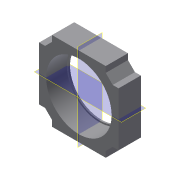
# Autodesk Inventor part: 20_Cube_Insert_VCM_MirrorMount_KES400A
Saved by Autodesk Inventor 2019.4 (Build 234330000, 330)
## iProperties
Created: 2019-10-23
Part Number: 20_Cube_Insert_VCM_MirrorMount_KES400A
Material: Generic
Document SubType Name: Modeling
Designer: marsikovabarbora
Density: 1 g/cm^3
Appearance: Default
Lens_diameter: 25,400 mm
Author: marsikovabarbora
Autodesk Inventor part; units mm, degrees
ref_plane "YZ Plane" through (0, 0, 0) normal (1, 0, 0) x (0, 1, 0)
ref_plane "XZ Plane" through (0, 0, 0) normal (0, 1, 0) x (-1, 0, 0)
ref_plane "XY Plane" through (0, 0, 0) normal (0, 0, 1) x (1, 0, 0)
sketch "Sketch1" plane through (0, 0, 0) normal (0, 0, 1) x (1, 0, 0)
  line L0 (-37.8611, 0) -> (52.8619, 0) construction
  line L1 (0, -34.8609) -> (0, 34.8609) construction
  line L2 (0, 0) -> (13.4339, 13.4339) construction
  line L3 (0, 0) -> (18.9985, 0) construction
  line L4 (0, 24.9006) -> (16.8, 24.9006)
  line L5 (16.8, 24.9006) -> (16.8, 21.2406)
  line L6 (16.8, 21.2406) -> (19.0203, 19.0203)
  line L7 (24.9006, 0) -> (24.9006, 16.8)
  line L8 (24.9006, 16.8) -> (21.2406, 16.8)
  line L9 (21.2406, 16.8) -> (19.0203, 19.0203)
  line L10 (0, 0) -> (-13.4339, 13.4339) construction
  line L11 (0, 0) -> (-18.9985, 0) construction
  line L12 (0, 24.9006) -> (-16.8, 24.9006)
  line L13 (-16.8, 24.9006) -> (-16.8, 21.2406)
  line L14 (-16.8, 21.2406) -> (-19.0203, 19.0203)
  line L15 (-24.9006, 0) -> (-24.9006, 16.8)
  line L16 (-24.9006, 16.8) -> (-21.2406, 16.8)
  line L17 (-21.2406, 16.8) -> (-19.0203, 19.0203)
  line L18 (0, 0) -> (13.4339, -13.4339) construction
  line L19 (0, -24.9006) -> (16.8, -24.9006)
  line L20 (16.8, -24.9006) -> (16.8, -21.2406)
  line L21 (16.8, -21.2406) -> (19.0203, -19.0203)
  line L22 (24.9006, 0) -> (24.9006, -16.8)
  line L23 (24.9006, -16.8) -> (21.2406, -16.8)
  line L24 (21.2406, -16.8) -> (19.0203, -19.0203)
  line L25 (0, 0) -> (-13.4339, -13.4339) construction
  line L26 (0, -24.9006) -> (-16.8, -24.9006)
  line L27 (-16.8, -24.9006) -> (-16.8, -21.2406)
  line L28 (-16.8, -21.2406) -> (-19.0203, -19.0203)
  line L29 (-24.9006, 0) -> (-24.9006, -16.8)
  line L30 (-24.9006, -16.8) -> (-21.2406, -16.8)
  line L31 (-21.2406, -16.8) -> (-19.0203, -19.0203)
  circle A0 centre (37.4, 10.6752) radius 1 projected
  circle A1 centre (30.9, -9.8248) radius 1 projected
  line L32 (39.9015, 13.4339) -> (24.9006, 13.4339)
  line L33 (24.9006, 13.4339) -> (24.9006, -12.4218)
  line L34 (24.9006, -12.4218) -> (39.9015, -12.4218)
  line L35 (39.9015, -12.4218) -> (39.9015, 13.4339)
  dimension "d0" = 45
  dimension "d1" = 3.14
  dimension "d2" = 3.66
  dimension "d3" = 16.8
  constraints: 68 end point, 24 symmetric about line, 6 point on line, 3 horizontal, 3 perpendicular, 2 parallel, 1 equal length
  measures "d0" angle of L3 L2
  measures "d1" distance of L5.end L6.end
  measures "d2" distance of L4.end L5.end
  measures "d3" distance of L4.start L4.end
extrude "Thickness" add sketch "Sketch1" along normal blind 14 contours L4 L5 L6 L9 L8 L7 L22 L23 L24 L21 L20 L19 L26 L27 L28 L31 L30 L29 L15 L16 L17 L14 L13 L12 | L32 L35 L34 L22 L7 | A0 | A1
sketch "Sketch3" plane through (0, 0, 0) normal (0, 0, -1) x (-1, 0, 0)
  line L0 (-16.8, 24.9006) -> (16.8, 24.9006) projected
  line L1 (16.8, 24.9006) -> (16.8, 21.2406) projected
  line L2 (16.8, 21.2406) -> (21.2406, 16.8) projected
  line L3 (21.2406, 16.8) -> (24.9006, 16.8) projected
  line L4 (24.9006, 16.8) -> (24.9006, -16.8) projected
  line L5 (24.9006, -16.8) -> (21.2406, -16.8) projected
  line L6 (21.2406, -16.8) -> (16.8, -21.2406) projected
  line L7 (16.8, -21.2406) -> (16.8, -24.9006) projected
  line L8 (16.8, -24.9006) -> (-16.8, -24.9006) projected
  line L9 (-16.8, -24.9006) -> (-16.8, -21.2406) projected
  line L10 (-16.8, -21.2406) -> (-21.2406, -16.8) projected
  line L11 (-21.2406, -16.8) -> (-24.9006, -16.8) projected
  line L12 (-24.9006, -16.8) -> (-24.9006, -12.4218) projected
  line L13 (-24.9006, 16.8) -> (-21.2406, 16.8) projected
  line L14 (-21.2406, 16.8) -> (-16.8, 21.2406) projected
  line L15 (-16.8, 21.2406) -> (-16.8, 24.9006) projected
  line L16 (16.8994, 25) -> (-16.8994, 25)
  line L17 (-16.8994, 25) -> (-16.8994, 21.2818)
  line L18 (-16.8994, 21.2818) -> (-21.2818, 16.8994)
  line L19 (-21.2818, 16.8994) -> (-25, 16.8994)
  line L20 (-25, 16.8994) -> (-25, -16.8994)
  line L21 (-25, -16.8994) -> (-21.2818, -16.8994)
  line L22 (-21.2818, -16.8994) -> (-16.8994, -21.2818)
  line L23 (-16.8994, -21.2818) -> (-16.8994, -25)
  line L24 (-16.8994, -25) -> (16.8994, -25)
  line L25 (16.8994, -25) -> (16.8994, -21.2818)
  line L26 (16.8994, -21.2818) -> (21.2818, -16.8994)
  line L27 (21.2818, -16.8994) -> (25, -16.8994)
  line L28 (25, -16.8994) -> (25, 16.8994)
  line L29 (25, 16.8994) -> (21.2818, 16.8994)
  line L30 (21.2818, 16.8994) -> (16.8994, 21.2818)
  line L31 (16.8994, 21.2818) -> (16.8994, 25)
  line L32 (-39.9015, 13.4339) -> (-24.9006, 13.4339) projected
  line L33 (-24.9006, 13.4339) -> (-24.9006, 16.8) projected
  line L34 (-24.9006, -12.4218) -> (-39.9015, -12.4218) projected
  line L35 (-39.9015, -12.4218) -> (-39.9015, 13.4339) projected
  point P0 (0, 0)
  dimension "d22" = 50
  constraints: 32 end point, 15 other
  measures "d22" distance between parallel lines of L20 L28
extrude "Extrusion3" add sketch "Sketch3" against normal up to surface (14 mm away)
ref_plane "Work Plane1" through (0, -16.8994, 0) normal (-1, 0, 0) x (0, 0, 1)
ref_plane "Work Plane2" through (-16.8994, 0, 0) normal (0, -1, 0) x (1, 0, 0)
sketch "Sketch4" plane through (0, 0, 0) normal (0, 0, -1) x (-1, 0, 0)
  arc A0 (12.7755, -29.7) -> (13.7755, -30.7) centre (13.7755, -29.7) ccw projected
  line L0 (13.7755, -30.7) -> (16.92, -30.7) projected
  line L1 (16.92, -30.7) -> (16.92, -5) projected
  line L2 (16.92, -5) -> (7.3923, -5) projected
  arc A1 (7.3923, -5) -> (6.3923, -6) centre (7.3923, -6) ccw projected
  line L3 (6.3923, -6) -> (6.3923, -7.8624) projected
  arc A2 (5.3923, -8.8624) -> (6.3923, -7.8624) centre (5.3923, -7.8624) ccw projected
  line L4 (5.3923, -8.8624) -> (-13.08, -8.8624) projected
  line L5 (-13.08, -8.8624) -> (-13.08, -20.397) projected
  arc A3 (-14.08, -21.397) -> (-13.08, -20.397) centre (-14.08, -20.397) ccw projected
  line L6 (-14.08, -21.397) -> (-15.08, -21.397) projected
  arc A4 (-15.08, -21.397) -> (-16.08, -22.397) centre (-15.08, -22.397) ccw projected
  line L7 (-16.08, -22.397) -> (-16.08, -24.9624) projected
  arc A5 (-16.08, -24.9624) -> (-15.08, -25.9624) centre (-15.08, -24.9624) ccw projected
  line L8 (-15.08, -25.9624) -> (11.7755, -25.9624) projected
  arc A6 (12.7755, -26.9624) -> (11.7755, -25.9624) centre (11.7755, -26.9624) ccw projected
  line L9 (12.7755, -26.9624) -> (12.7755, -29.7) projected
  line L10 (4.42, -24) -> (-11.08, -24) projected
  line L11 (-11.08, -24) -> (-11.08, -10.5) projected
  line L12 (-11.08, -10.5) -> (4.42, -10.5) projected
  line L13 (4.42, -10.5) -> (4.42, -24) projected
  circle A7 centre (14.42, -28) radius 1 projected
  circle A8 centre (7.92, -7.5) radius 1 projected
  circle A9 centre (-13.58, -23) radius 1 projected
  arc A10 (12.7755, 5.3) -> (13.7755, 4.3) centre (13.7755, 5.3) ccw projected
  line L14 (13.7755, 4.3) -> (16.92, 4.3) projected
  line L15 (16.92, 4.3) -> (16.92, 30) projected
  line L16 (16.92, 30) -> (7.3923, 30) projected
  arc A11 (7.3923, 30) -> (6.3923, 29) centre (7.3923, 29) ccw projected
  line L17 (6.3923, 29) -> (6.3923, 27.1376) projected
  arc A12 (5.3923, 26.1376) -> (6.3923, 27.1376) centre (5.3923, 27.1376) ccw projected
  line L18 (5.3923, 26.1376) -> (-13.08, 26.1376) projected
  line L19 (-13.08, 26.1376) -> (-13.08, 14.603) projected
  arc A13 (-14.08, 13.603) -> (-13.08, 14.603) centre (-14.08, 14.603) ccw projected
  line L20 (-14.08, 13.603) -> (-15.08, 13.603) projected
  arc A14 (-15.08, 13.603) -> (-16.08, 12.603) centre (-15.08, 12.603) ccw projected
  line L21 (-16.08, 12.603) -> (-16.08, 10.0376) projected
  arc A15 (-16.08, 10.0376) -> (-15.08, 9.0376) centre (-15.08, 10.0376) ccw projected
  line L22 (-15.08, 9.0376) -> (11.7755, 9.0376) projected
  arc A16 (12.7755, 8.0376) -> (11.7755, 9.0376) centre (11.7755, 8.0376) ccw projected
  line L23 (12.7755, 8.0376) -> (12.7755, 5.3) projected
  line L24 (4.42, 11) -> (-11.08, 11) projected
  line L25 (-11.08, 11) -> (-11.08, 24.5) projected
  line L26 (-11.08, 24.5) -> (4.42, 24.5) projected
  line L27 (4.42, 24.5) -> (4.42, 11) projected
  circle A17 centre (14.42, 7) radius 1 projected
  circle A18 centre (7.92, 27.5) radius 1 projected
  circle A19 centre (-13.58, 12) radius 1 projected
  arc A20 (-35.7555, 12.3752) -> (-36.7555, 13.3752) centre (-36.7555, 12.3752) ccw projected
  line L28 (-36.7555, 13.3752) -> (-39.9, 13.3752) projected
  line L29 (-39.9, 13.3752) -> (-39.9, -12.3248) projected
  line L30 (-39.9, -12.3248) -> (-30.3723, -12.3248) projected
  arc A21 (-30.3723, -12.3248) -> (-29.3723, -11.3248) centre (-30.3723, -11.3248) ccw projected
  line L31 (-29.3723, -11.3248) -> (-29.3723, -9.4624) projected
  arc A22 (-28.3723, -8.4624) -> (-29.3723, -9.4624) centre (-28.3723, -9.4624) ccw projected
  line L32 (-28.3723, -8.4624) -> (-9.9, -8.4624) projected
  line L33 (-9.9, -8.4624) -> (-9.9, 3.0723) projected
  arc A23 (-8.9, 4.0723) -> (-9.9, 3.0723) centre (-8.9, 3.0723) ccw projected
  line L34 (-8.9, 4.0723) -> (-7.9, 4.0723) projected
  arc A24 (-7.9, 4.0723) -> (-6.9, 5.0723) centre (-7.9, 5.0723) ccw projected
  line L35 (-6.9, 5.0723) -> (-6.9, 7.6376) projected
  arc A25 (-6.9, 7.6376) -> (-7.9, 8.6376) centre (-7.9, 7.6376) ccw projected
  line L36 (-7.9, 8.6376) -> (-34.7555, 8.6376) projected
  arc A26 (-35.7555, 9.6376) -> (-34.7555, 8.6376) centre (-34.7555, 9.6376) ccw projected
  line L37 (-35.7555, 9.6376) -> (-35.7555, 12.3752) projected
  line L38 (-27.4, 6.6752) -> (-11.9, 6.6752) projected
  line L39 (-11.9, 6.6752) -> (-11.9, -6.8248) projected
  line L40 (-11.9, -6.8248) -> (-27.4, -6.8248) projected
  line L41 (-27.4, -6.8248) -> (-27.4, 6.6752) projected
  circle A27 centre (-37.4, 10.6752) radius 1 projected
  circle A28 centre (-30.9, -9.8248) radius 1 projected
  circle A29 centre (-9.4, 5.6752) radius 1 projected
  point P0 (0, 0)
hole "Hole2" at (-7.92, -7.5, 0) at (-14.42, 7, 0) at (13.58, 12, 0) at (9.4, 5.6752, 0) at (30.9, -9.8248, 0) at (37.4, 10.6752, 0) direction (0, 0, 1) diameter 1.8 end through all
equation "\"Lens_diameter\" = 25.4"
body "Solid1"
